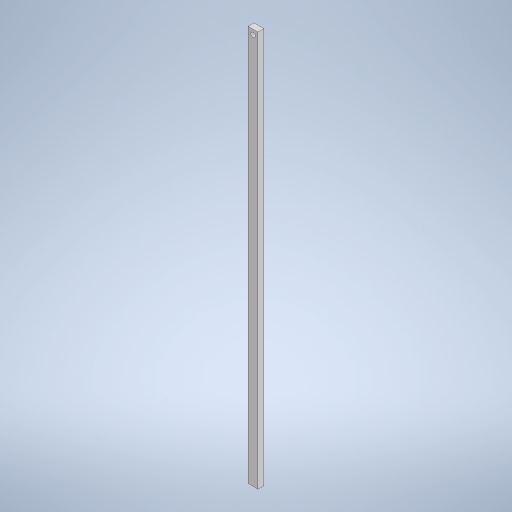
# Autodesk Inventor part: Tx_fixed_stick
Saved by Autodesk Inventor 2023 (Build 270158000, 158)
## iProperties
Created: 2023-09-18
Part Number: Tx_fixed_stick
Material: 一般
Document SubType Name: Modeling
Designer: 310611102
Density: 1 g/cm^3
Appearance: 預設
Author: 310611102
Autodesk Inventor part; units mm, degrees
ref_plane "YZ Plane" through (0, 0, 0) normal (1, 0, 0) x (0, 1, 0)
ref_plane "XZ Plane" through (0, 0, 0) normal (0, 1, 0) x (-1, 0, 0)
ref_plane "XY Plane" through (0, 0, 0) normal (0, 0, 1) x (1, 0, 0)
sketch "Sketch1" plane through (0, 0, 0) normal (0, 0, 1) x (1, 0, 0)
  line L0 (-5, -200) -> (5, -200)
  line L1 (5, -200) -> (5, 200)
  line L2 (5, 200) -> (-5, 200)
  line L3 (-5, 200) -> (-5, -200)
  line L4 (-5, -200) -> (5, 200) construction
  line L5 (5, -200) -> (-5, 200) construction
  circle A0 centre (0, 195) radius 2.25
  point P0 (0, 0)
  point P1 (0, 200)
  dimension "d0" = 10
  dimension "d1" = 400
  dimension "d2" = 4.5
  dimension "d3" = 5
  constraints: 12 end point, 3 midpoint, 2 parallel, 1 centre point, 1 horizontal, 1 perpendicular, 1 vertical alignment
  measures "d0" distance of L1.end L2.end
  measures "d1" distance of L0.end L1.end
  measures "d2" diameter of A0
  measures "d3" distance from line of L2 A0.centre
extrude "Extrusion1" add sketch "Sketch1" along normal blind 6
body "Solid1"
